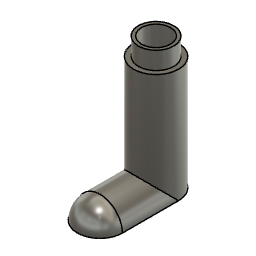
leg_V1 v2 (Autodesk Fusion 360 design; units mm, degrees)
Autodesk Fusion 360 part; units mm, degrees
cylinder "CylinderPrimitive1" add diameter 28 height 71 placed x (1, 0, 0) y (0, 0, -1) z (0, 1, 0) at (0, 0, 0) makes body 1
cylinder "CylinderPrimitive2" add diameter 22 height 82 placed x (1, 0, 0) y (0, 0, -1) z (0, 1, 0) at (0, 0, 0) bodies 1
hole "Hole1" at (0, 82, 0) direction (0, -1, 0) diameter 18 end through all bodies 1
cylinder "CylinderPrimitive3" add diameter 28 height 35 placed x (1, 0, 0) y (0, 1, 0) z (0, 0, 1) at (0, 0, 0) bodies 1
box "BoxPrimitive1" add length 16 width 90 height 32 placed x (0, 1, 0) y (0, 0, 1) z (1, 0, 0) at (0, -16, -11) separate body makes body 2
move_body "Move1" bodies 2 to x (1, 0, 0) y (0, 1, 0) z (0, 0, 1) at (-16, 0, 0)
sphere "SpherePrimitive1" add diameter 28 placed x (1, 0, 0) y (0, 1, 0) z (0, 0, 1) at (0, 0, 35) bodies 1
combine "Combine1" operation cut target body 1 tool bodies 2
hole "Hole2" at (0, 0, 0) direction (0, 1, 0) diameter 19 depth 15 tip angle 118 bodies 1
hole "Hole3" at (0.1519, 0, 30.6055) direction (0, 1, 0) diameter 1.623 depth 6 tip angle 118 counterbore diameter 2 counterbore depth 1 bodies 1
